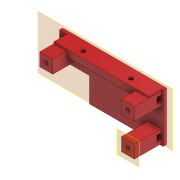
# Autodesk Inventor part: spacer for new drivetrain 2 top
Saved by Autodesk Inventor 2020 (Build 240168000, 168)
## iProperties
Created: 2020-02-19
Part Number: spacer for new drivetrain 2 top
Material: Generic
Document SubType Name: Modeling
Designer: jackm
Density: 1 g/cm^3
Appearance: Default
Author: jackm
Autodesk Inventor part; units mm, degrees
ref_plane "YZ Plane" through (0, 0, 0) normal (1, 0, 0) x (0, 1, 0)
ref_plane "XZ Plane" through (0, 0, 0) normal (0, 1, 0) x (-1, 0, 0)
ref_plane "XY Plane" through (0, 0, 0) normal (0, 0, 1) x (1, 0, 0)
ref_plane "Work Plane1" through (0, 0, 0) normal (0, 0, 1) x (1, 0, 0)
sketch "Sketch1" plane through (0, 0, 0) normal (0, 0, 1) x (1, 0, 0)
  line L0 (120, 0) -> (120, 48) construction
  line L1 (0, 48) -> (120, 48) construction
  line L2 (0, 0) -> (0, 48) construction
  line L3 (0, 0) -> (120, 0) construction
  circle A0 centre (96, 24) radius 7 construction
  circle A1 centre (72, 24) radius 7 construction
  arc A2 (88.9289, 33.8995) -> (86.1005, 31.0711) centre (87.5147, 32.4853) ccw construction
  line L4 (89.4142, 33.4142) -> (88.9289, 33.8995) construction
  arc A3 (86.5858, 30.5858) -> (89.4142, 33.4142) centre (88, 32) ccw construction
  line L5 (86.1005, 31.0711) -> (86.5858, 30.5858) construction
  line L6 (83.3137, 22) -> (84.6863, 22) construction
  arc A4 (83.3137, 26) -> (83.3137, 22) centre (83.3137, 24) ccw construction
  line L7 (84.6863, 26) -> (83.3137, 26) construction
  arc A5 (84.6863, 22) -> (84.6863, 26) centre (84.6863, 24) ccw construction
  arc A6 (86.1005, 16.9289) -> (88.9289, 14.1005) centre (87.5147, 15.5147) ccw construction
  line L8 (86.5858, 17.4142) -> (86.1005, 16.9289) construction
  arc A7 (89.4142, 14.5858) -> (86.5858, 17.4142) centre (88, 16) ccw construction
  line L9 (88.9289, 14.1005) -> (89.4142, 14.5858) construction
  arc A8 (105.8995, 31.0711) -> (103.0711, 33.8995) centre (104.4853, 32.4853) ccw construction
  line L10 (105.4142, 30.5858) -> (105.8995, 31.0711) construction
  arc A9 (102.5858, 33.4142) -> (105.4142, 30.5858) centre (104, 32) ccw construction
  line L11 (103.0711, 33.8995) -> (102.5858, 33.4142) construction
  line L12 (108.6863, 26) -> (107.3137, 26) construction
  arc A10 (108.6863, 22) -> (108.6863, 26) centre (108.6863, 24) ccw construction
  line L13 (107.3137, 22) -> (108.6863, 22) construction
  arc A11 (107.3137, 26) -> (107.3137, 22) centre (107.3137, 24) ccw construction
  line L14 (98, 35.3137) -> (98, 40) construction
  arc A12 (94, 35.3137) -> (98, 35.3137) centre (96, 35.3137) ccw construction
  line L15 (94, 40) -> (94, 35.3137) construction
  arc A13 (98, 40) -> (94, 40) centre (96, 40) ccw construction
  circle A14 centre (88, 40) radius 2 construction
  circle A15 centre (80, 40) radius 2 construction
  line L16 (74, 35.3137) -> (74, 40) construction
  arc A16 (70, 35.3137) -> (74, 35.3137) centre (72, 35.3137) ccw construction
  line L17 (70, 40) -> (70, 35.3137) construction
  arc A17 (74, 40) -> (70, 40) centre (72, 40) ccw construction
  circle A18 centre (64, 40) radius 2 construction
  circle A19 centre (56, 40) radius 2 construction
  line L18 (50, 35.3137) -> (50, 40) construction
  arc A20 (46, 35.3137) -> (50, 35.3137) centre (48, 35.3137) ccw construction
  line L19 (46, 40) -> (46, 35.3137) construction
  arc A21 (50, 40) -> (46, 40) centre (48, 40) ccw construction
  circle A22 centre (40, 40) radius 2 construction
  circle A23 centre (32, 40) radius 2 construction
  line L20 (26, 35.3137) -> (26, 40) construction
  arc A24 (22, 35.3137) -> (26, 35.3137) centre (24, 35.3137) ccw construction
  line L21 (22, 40) -> (22, 35.3137) construction
  arc A25 (26, 40) -> (22, 40) centre (24, 40) ccw construction
  circle A26 centre (16, 40) radius 2 construction
  circle A27 centre (8, 40) radius 2 construction
  line L22 (94, 12.6863) -> (94, 8) construction
  arc A28 (98, 12.6863) -> (94, 12.6863) centre (96, 12.6863) ccw construction
  line L23 (98, 8) -> (98, 12.6863) construction
  arc A29 (94, 8) -> (98, 8) centre (96, 8) ccw construction
  circle A30 centre (88, 8) radius 2 construction
  circle A31 centre (80, 8) radius 2 construction
  line L24 (70, 12.6863) -> (70, 8) construction
  arc A32 (74, 12.6863) -> (70, 12.6863) centre (72, 12.6863) ccw construction
  line L25 (74, 8) -> (74, 12.6863) construction
  arc A33 (70, 8) -> (74, 8) centre (72, 8) ccw construction
  circle A34 centre (64, 8) radius 2 construction
  circle A35 centre (56, 8) radius 2 construction
  line L26 (46, 12.6863) -> (46, 8) construction
  arc A36 (50, 12.6863) -> (46, 12.6863) centre (48, 12.6863) ccw construction
  line L27 (50, 8) -> (50, 12.6863) construction
  arc A37 (46, 8) -> (50, 8) centre (48, 8) ccw construction
  circle A38 centre (40, 8) radius 2 construction
  circle A39 centre (32, 8) radius 2 construction
  line L28 (22, 12.6863) -> (22, 8) construction
  arc A40 (26, 12.6863) -> (22, 12.6863) centre (24, 12.6863) ccw construction
  line L29 (26, 8) -> (26, 12.6863) construction
  arc A41 (22, 8) -> (26, 8) centre (24, 8) ccw construction
  circle A42 centre (16, 8) radius 2 construction
  circle A43 centre (8, 8) radius 2 construction
  arc A44 (9.8995, 31.0711) -> (7.0711, 33.8995) centre (8.4853, 32.4853) ccw construction
  line L30 (9.4142, 30.5858) -> (9.8995, 31.0711) construction
  arc A45 (6.5858, 33.4142) -> (9.4142, 30.5858) centre (8, 32) ccw construction
  line L31 (7.0711, 33.8995) -> (6.5858, 33.4142) construction
  arc A46 (7.0711, 14.1005) -> (9.8995, 16.9289) centre (8.4853, 15.5147) ccw construction
  line L32 (6.5858, 14.5858) -> (7.0711, 14.1005) construction
  arc A47 (9.4142, 17.4142) -> (6.5858, 14.5858) centre (8, 16) ccw construction
  line L33 (9.8995, 16.9289) -> (9.4142, 17.4142) construction
  arc A48 (112.9289, 33.8995) -> (110.1005, 31.0711) centre (111.5147, 32.4853) ccw construction
  line L34 (113.4142, 33.4142) -> (112.9289, 33.8995) construction
  arc A49 (110.5858, 30.5858) -> (113.4142, 33.4142) centre (112, 32) ccw construction
  line L35 (110.1005, 31.0711) -> (110.5858, 30.5858) construction
  arc A50 (110.1005, 16.9289) -> (112.9289, 14.1005) centre (111.5147, 15.5147) ccw construction
  line L36 (110.5858, 17.4142) -> (110.1005, 16.9289) construction
  arc A51 (113.4142, 14.5858) -> (110.5858, 17.4142) centre (112, 16) ccw construction
  line L37 (112.9289, 14.1005) -> (113.4142, 14.5858) construction
  circle A52 centre (104, 8) radius 2 construction
  circle A53 centre (104, 40) radius 2 construction
  circle A54 centre (112, 40) radius 2 construction
  circle A55 centre (112, 8) radius 2 construction
  arc A56 (33.8995, 31.0711) -> (31.0711, 33.8995) centre (32.4853, 32.4853) ccw construction
  line L38 (33.4142, 30.5858) -> (33.8995, 31.0711) construction
  arc A57 (30.5858, 33.4142) -> (33.4142, 30.5858) centre (32, 32) ccw construction
  line L39 (31.0711, 33.8995) -> (30.5858, 33.4142) construction
  arc A58 (57.8995, 31.0711) -> (55.0711, 33.8995) centre (56.4853, 32.4853) ccw construction
  line L40 (57.4142, 30.5858) -> (57.8995, 31.0711) construction
  arc A59 (54.5858, 33.4142) -> (57.4142, 30.5858) centre (56, 32) ccw construction
  line L41 (55.0711, 33.8995) -> (54.5858, 33.4142) construction
  arc A60 (81.8995, 31.0711) -> (79.0711, 33.8995) centre (80.4853, 32.4853) ccw construction
  line L42 (81.4142, 30.5858) -> (81.8995, 31.0711) construction
  arc A61 (78.5858, 33.4142) -> (81.4142, 30.5858) centre (80, 32) ccw construction
  line L43 (79.0711, 33.8995) -> (78.5858, 33.4142) construction
  arc A62 (14.1005, 16.9289) -> (16.9289, 14.1005) centre (15.5147, 15.5147) ccw construction
  line L44 (14.5858, 17.4142) -> (14.1005, 16.9289) construction
  arc A63 (17.4142, 14.5858) -> (14.5858, 17.4142) centre (16, 16) ccw construction
  line L45 (16.9289, 14.1005) -> (17.4142, 14.5858) construction
  arc A64 (38.1005, 16.9289) -> (40.9289, 14.1005) centre (39.5147, 15.5147) ccw construction
  line L46 (38.5858, 17.4142) -> (38.1005, 16.9289) construction
  arc A65 (41.4142, 14.5858) -> (38.5858, 17.4142) centre (40, 16) ccw construction
  line L47 (40.9289, 14.1005) -> (41.4142, 14.5858) construction
  arc A66 (62.1005, 16.9289) -> (64.9289, 14.1005) centre (63.5147, 15.5147) ccw construction
  line L48 (62.5858, 17.4142) -> (62.1005, 16.9289) construction
  arc A67 (65.4142, 14.5858) -> (62.5858, 17.4142) centre (64, 16) ccw construction
  line L49 (64.9289, 14.1005) -> (65.4142, 14.5858) construction
  line L50 (11.3137, 22) -> (12.6863, 22) construction
  arc A68 (11.3137, 26) -> (11.3137, 22) centre (11.3137, 24) ccw construction
  line L51 (12.6863, 26) -> (11.3137, 26) construction
  arc A69 (12.6863, 22) -> (12.6863, 26) centre (12.6863, 24) ccw construction
  line L52 (35.3137, 22) -> (36.6863, 22) construction
  arc A70 (35.3137, 26) -> (35.3137, 22) centre (35.3137, 24) ccw construction
  line L53 (36.6863, 26) -> (35.3137, 26) construction
  arc A71 (36.6863, 22) -> (36.6863, 26) centre (36.6863, 24) ccw construction
  line L54 (59.3137, 22) -> (60.6863, 22) construction
  arc A72 (59.3137, 26) -> (59.3137, 22) centre (59.3137, 24) ccw construction
  line L55 (60.6863, 26) -> (59.3137, 26) construction
  arc A73 (60.6863, 22) -> (60.6863, 26) centre (60.6863, 24) ccw construction
  arc A74 (16.9289, 33.8995) -> (14.1005, 31.0711) centre (15.5147, 32.4853) ccw construction
  line L56 (17.4142, 33.4142) -> (16.9289, 33.8995) construction
  arc A75 (14.5858, 30.5858) -> (17.4142, 33.4142) centre (16, 32) ccw construction
  line L57 (14.1005, 31.0711) -> (14.5858, 30.5858) construction
  arc A76 (40.9289, 33.8995) -> (38.1005, 31.0711) centre (39.5147, 32.4853) ccw construction
  line L58 (41.4142, 33.4142) -> (40.9289, 33.8995) construction
  arc A77 (38.5858, 30.5858) -> (41.4142, 33.4142) centre (40, 32) ccw construction
  line L59 (38.1005, 31.0711) -> (38.5858, 30.5858) construction
  arc A78 (64.9289, 33.8995) -> (62.1005, 31.0711) centre (63.5147, 32.4853) ccw construction
  line L60 (65.4142, 33.4142) -> (64.9289, 33.8995) construction
  arc A79 (62.5858, 30.5858) -> (65.4142, 33.4142) centre (64, 32) ccw construction
  line L61 (62.1005, 31.0711) -> (62.5858, 30.5858) construction
  arc A80 (31.0711, 14.1005) -> (33.8995, 16.9289) centre (32.4853, 15.5147) ccw construction
  line L62 (30.5858, 14.5858) -> (31.0711, 14.1005) construction
  arc A81 (33.4142, 17.4142) -> (30.5858, 14.5858) centre (32, 16) ccw construction
  line L63 (33.8995, 16.9289) -> (33.4142, 17.4142) construction
  arc A82 (55.0711, 14.1005) -> (57.8995, 16.9289) centre (56.4853, 15.5147) ccw construction
  line L64 (54.5858, 14.5858) -> (55.0711, 14.1005) construction
  arc A83 (57.4142, 17.4142) -> (54.5858, 14.5858) centre (56, 16) ccw construction
  line L65 (57.8995, 16.9289) -> (57.4142, 17.4142) construction
  arc A84 (79.0711, 14.1005) -> (81.8995, 16.9289) centre (80.4853, 15.5147) ccw construction
  line L66 (78.5858, 14.5858) -> (79.0711, 14.1005) construction
  arc A85 (81.4142, 17.4142) -> (78.5858, 14.5858) centre (80, 16) ccw construction
  line L67 (81.8995, 16.9289) -> (81.4142, 17.4142) construction
  arc A86 (103.0711, 14.1005) -> (105.8995, 16.9289) centre (104.4853, 15.5147) ccw construction
  line L68 (102.5858, 14.5858) -> (103.0711, 14.1005) construction
  arc A87 (105.4142, 17.4142) -> (102.5858, 14.5858) centre (104, 16) ccw construction
  line L69 (105.8995, 16.9289) -> (105.4142, 17.4142) construction
  circle A88 centre (24, 24) radius 7 construction
  circle A89 centre (48, 24) radius 7 construction
  line L70 (120, 0) -> (48, 0)
  line L71 (18.4, 19.8) -> (18.4, 48)
  line L72 (18.4, 48) -> (120, 48)
  line L73 (120, 0) -> (120, 48)
  line L74 (18.4, 24) -> (48, 24)
  line L75 (48, 24) -> (48, 0)
  point P0 (18.4, 0)
  dimension "d0" = 101.6
  constraints: 12 end point, 4 perpendicular, 3 point on line, 1 collinear, 2 other
  measures "d0" distance of L0.start point (18.4, 0)
extrude "Extrusion1" add sketch "Sketch1" along normal blind 3.175
ref_plane "Work Plane2" through (112, 8, 29.6672) normal (0, 0, 1) x (1, 0, 0)
sketch "Sketch5" plane through (112, 8, 29.6672) normal (0, 0, 1) x (1, 0, 0)
  circle A0 centre (0, 0) radius 3.81 construction
  circle A1 centre (0, 32) radius 3.81 construction
  circle A2 centre (-80, 32) radius 3.81 construction
  circle A3 centre (-80, 0) radius 3.81 construction
  circle A4 centre (0, 0) radius 1.9304
  circle A5 centre (0, 32) radius 1.9304
  circle A6 centre (-80, 0) radius 1.9304
  circle A7 centre (-80, 32) radius 1.9304
  point P0 (-112, -8)
  dimension "d25" = 3.8608
  dimension "d26" = 3.8608
  dimension "d27" = 3.8608
  dimension "d28" = 3.8608
  constraints: 4 centre point, 4 coincident
  measures "d25" diameter of A4
  measures "d26" diameter of A5
  measures "d27" diameter of A6
  measures "d28" diameter of A7
extrude "Extrusion4" cut sketch "Sketch5" against normal through all
sketch "Sketch6" plane through (0, 0, 3.175) normal (0, 0, 1) x (1, 0, 0)
  circle A0 centre (112, 40) radius 1.9304 projected
  line L0 (120, 0) -> (120, 48) projected
  line L1 (112, 42.9845) -> (124.5106, 42.9845) construction
  line L2 (112, 37.0028) -> (120.8332, 37.0028) construction
  line L3 (112, 40) -> (108.547, 40.0987)
  line L4 (108.547, 40.0987) -> (109.8492, 37.8432)
  line L5 (108.547, 40.0987) -> (111.1514, 40.0987) construction
  line L6 (109.8492, 37.8432) -> (110.3344, 37.0028)
  line L7 (108.547, 40.0987) -> (110.2132, 42.9845)
  line L8 (108.547, 40.0987) -> (114.1138, 40.0987) construction
  line L9 (110.2132, 42.9845) -> (118.2904, 42.9845)
  line L10 (110.3344, 37.0028) -> (118.2904, 37.0028)
  line L11 (118.2904, 46.3436) -> (105.5904, 46.3436)
  line L12 (105.5904, 46.3436) -> (105.5904, 33.6436)
  line L13 (105.5904, 33.6436) -> (118.2904, 33.6436)
  line L14 (118.2904, 33.6436) -> (118.2904, 37.0028)
  line L15 (118.2904, 46.3436) -> (118.2904, 42.9845)
  circle A1 centre (112, 8) radius 1.9304 construction
  line L16 (112, 10.9845) -> (124.5106, 10.9845) construction
  line L17 (112, 5.0028) -> (120.8332, 5.0028) construction
  line L18 (112, 8) -> (108.547, 8.0987)
  line L19 (108.547, 8.0987) -> (109.8492, 5.8432)
  line L20 (108.547, 8.0987) -> (111.1514, 8.0987) construction
  line L21 (109.8492, 5.8432) -> (110.3344, 5.0028)
  line L22 (108.547, 8.0987) -> (110.2132, 10.9845)
  line L23 (108.547, 8.0987) -> (114.1138, 8.0987) construction
  line L24 (110.2132, 10.9845) -> (118.2904, 10.9845)
  line L25 (110.3344, 5.0028) -> (118.2904, 5.0028)
  line L26 (118.2904, 14.3436) -> (105.5904, 14.3436)
  line L27 (105.5904, 14.3436) -> (105.5904, 1.6436)
  line L28 (105.5904, 1.6436) -> (118.2904, 1.6436)
  line L29 (118.2904, 1.6436) -> (118.2904, 5.0028)
  line L30 (118.2904, 14.3436) -> (118.2904, 10.9845)
  circle A2 centre (32, 40) radius 1.9304 construction
  line L31 (32.0099, 37.0155) -> (19.4993, 36.974) construction
  line L32 (31.9901, 42.9972) -> (23.1569, 42.9679) construction
  line L33 (32, 40) -> (35.4533, 39.9128)
  line L34 (35.4533, 39.9128) -> (34.1437, 42.1639)
  line L35 (35.4533, 39.9128) -> (32.849, 39.9042) construction
  line L36 (34.1437, 42.1639) -> (33.6557, 43.0027)
  line L37 (35.4533, 39.9128) -> (33.7967, 37.0214)
  line L38 (35.4533, 39.9128) -> (29.8865, 39.8943) construction
  line L39 (33.7967, 37.0214) -> (25.7196, 36.9947)
  line L40 (33.6557, 43.0027) -> (25.6997, 42.9763)
  line L41 (25.7307, 33.6355) -> (38.4306, 33.6776)
  line L42 (38.4306, 33.6776) -> (38.3885, 46.3776)
  line L43 (38.3885, 46.3776) -> (25.6886, 46.3355)
  line L44 (25.6886, 46.3355) -> (25.6997, 42.9763)
  line L45 (25.7307, 33.6355) -> (25.7196, 36.9947)
  point P0 (0, 0)
  dimension "d32" = 2.9845
  dimension "d33" = 2.9972
  dimension "d36" = 3.4544
  dimension "d37" = 60
  dimension "d38" = 60
  dimension "d39" = 8.0772
  dimension "d41" = 12.7
  dimension "d42" = 12.7
  dimension "d43" = 12.7
  dimension "d44" = 2.9845
  dimension "d45" = 2.9972
  dimension "d46" = 3.4544
  dimension "d47" = 60
  dimension "d48" = 60
  dimension "d49" = 8.0772
  dimension "d50" = 12.7
  dimension "d51" = 12.7
  dimension "d52" = 12.7
  dimension "d69" = 2.9845
  dimension "d70" = 2.9972
  dimension "d71" = 3.4544
  dimension "d72" = 60
  dimension "d73" = 60
  dimension "d74" = 8.0772
  dimension "d75" = 12.7
  dimension "d76" = 12.7
  dimension "d77" = 12.7
  constraints: 90 end point, 9 point on line, 8 horizontal, 6 perpendicular, 3 equal length
  measures "d32" distance of L3.start L1.start
  measures "d33" distance of L3.start L2.start
  measures "d36" distance of L3.start L3.end
  measures "d37" angle of L4 L5
  measures "d38" angle of L8 L7
  measures "d39" distance of L7.end L9.end
  measures "d41" distance of L11.start L11.end
  measures "d42" distance of L11.end L12.end
  measures "d43" distance of L12.end L13.end
  measures "d44" distance of L18.start L16.start
  measures "d45" distance of L18.start L17.start
  measures "d46" distance of L18.start L23.start
  measures "d47" angle of L19 L20
  measures "d48" angle of L23 L22
  measures "d49" distance of L22.end L30.end
  measures "d50" distance of L26.start L27.start
  measures "d51" distance of L27.start L28.start
  measures "d52" distance of L28.start L28.end
  measures "d69" distance of L33.start L31.start
  measures "d70" distance of L33.start L32.start
  measures "d71" distance of L33.start L35.start
  measures "d72" angle of L34 L35
  measures "d73" angle of L38 L37
  measures "d74" distance of L37.end L39.end
  measures "d75" distance of L45.start L41.end
  measures "d76" distance of L41.end L43.start
  measures "d77" distance of L43.start L43.end
extrude "Extrusion5" add sketch "Sketch6" along normal blind 4.3942 contours L4 L6 L10 L14 L13 L12 L11 L15 L9 L7 | L19 L21 L25 L29 L28 L27 L26 L30 L24 L22 | L34 L36 L40 L44 L43 L42 L41 L45 L39 L37
sketch "Sketch7" plane through (0, 0, 7.5692) normal (0, 0, 1) x (1, 0, 0)
  line L0 (105.5904, 33.6436) -> (105.5904, 46.3436) projected
  line L1 (118.2904, 46.3436) -> (118.2904, 42.9845) projected
  line L2 (105.5904, 46.3436) -> (118.2904, 46.3436)
  line L3 (118.2904, 37.0028) -> (118.2904, 33.6436) projected
  line L4 (118.2904, 46.3436) -> (118.2904, 33.6436)
  line L5 (118.2904, 33.6436) -> (105.5904, 33.6436) projected
  line L6 (118.2904, 33.6436) -> (105.5904, 33.6436)
  line L7 (105.5904, 33.6436) -> (105.5904, 46.3436)
  line L8 (105.5904, 14.3436) -> (105.5904, 1.6436) projected
  line L9 (118.2904, 14.3436) -> (118.2904, 10.9845) projected
  line L10 (105.5904, 14.3436) -> (118.2904, 14.3436)
  line L11 (118.2904, 14.3436) -> (118.2904, 1.6436)
  line L12 (105.5904, 1.6436) -> (118.2904, 1.6436) projected
  line L13 (118.2904, 1.6436) -> (105.5904, 1.6436)
  line L14 (105.5904, 1.6436) -> (105.5904, 14.3436)
  line L15 (25.6886, 46.3355) -> (38.3885, 46.3776) projected
  line L16 (38.4306, 33.6776) -> (38.3885, 46.3776) projected
  line L17 (25.6886, 46.3355) -> (38.3885, 46.3776)
  line L18 (38.3885, 46.3776) -> (38.4306, 33.6776)
  line L19 (38.4306, 33.6776) -> (25.7307, 33.6355) projected
  line L20 (38.4306, 33.6776) -> (25.7307, 33.6355)
  line L21 (25.6886, 46.3355) -> (25.6997, 42.9763) projected
  line L22 (25.7307, 33.6355) -> (25.6886, 46.3355)
  point P0 (0, 0)
  point P1 (25.6487, 46.2826)
  point P2 (25.6642, 33.5826)
  point P3 (38.3487, 46.2981)
  point P4 (38.3642, 33.5981)
  constraints: 24 end point, 5 perpendicular, 4 collinear, 2 horizontal
extrude "Extrusion6" add sketch "Sketch7" along normal blind 22.098
sketch "Sketch8" plane through (0, 0, 29.6672) normal (0, 0, 1) x (1, 0, 0)
  circle A0 centre (32, 40) radius 1.9304 construction
  circle A1 centre (112, 40) radius 1.9304 construction
  circle A2 centre (112, 8) radius 1.9304 construction
  circle A3 centre (32, 40) radius 1.9304 projected
  circle A4 centre (32, 40) radius 1.9304
  circle A5 centre (112, 40) radius 1.9304 projected
  circle A6 centre (112, 40) radius 1.9304
  circle A7 centre (112, 8) radius 1.9304 projected
  circle A8 centre (112, 8) radius 1.9304
  point P0 (0, 0)
  constraints: 3 centre point, 3 coincident
extrude "Extrusion7" cut sketch "Sketch8" against normal through all
sketch "Sketch9" plane through (18.4, 48, 0) normal (0, 1, 0) x (1, 0, 0)
  line L0 (7.3196, -3.175) -> (7.3196, -7.5692) projected
  line L1 (99.8904, -3.175) -> (99.8904, -29.6672) projected
  line L2 (7.3196, -3.175) -> (99.8904, -3.175)
  line L3 (99.8904, -3.175) -> (99.8904, -15.875)
  line L4 (99.8904, -15.875) -> (7.3196, -15.875)
  line L5 (7.3196, -15.875) -> (7.3196, -3.175)
  point P0 (-18.4, 0)
  point P1 (7.3196, -7.5692)
  dimension "d78" = 12.7
  constraints: 8 end point, 2 parallel, 1 horizontal, 1 perpendicular, 1 point on line
  measures "d78" distance of L2.end L3.end
extrude "Extrusion8" add sketch "Sketch9" against normal up to surface surface through (38.3885, 46.3776, 3.175) normal (-0.0033161, 0.9999945, 0)
sketch "Sketch10" plane through (38.3885, 46.3776, 3.175) normal (0.0033161, -0.9999945, 0) x (0.9999945, 0.0033161, 0)
  line L0 (79.9023, 12.7) -> (0, 12.7) projected
  line L1 (67.1592, 0) -> (67.1592, 26.4922) projected
  line L2 (0, 12.7) -> (67.1592, 12.7)
  line L3 (67.1592, 12.7) -> (67.1592, 0)
  line L4 (67.1592, 0) -> (0, 0)
  line L5 (0, 0) -> (0, 12.7)
  point P0 (-38.5421, -3.175)
  constraints: 8 end point, 2 parallel, 1 horizontal, 1 perpendicular
extrude "Extrusion9" add sketch "Sketch10" along normal blind 5.08
sketch "Sketch11" plane through (38.4054, 41.2976, 3.175) normal (0.0033161, -0.9999945, 0) x (0.9999945, 0.0033161, 0)
  circle A0 centre (9.632, 6.2821) radius 4.6609 construction
  line L0 (14.2929, 6.2821) -> (11.9624, 10.3186)
  line L1 (11.9624, 10.3186) -> (7.3015, 10.3186)
  line L2 (7.3015, 10.3186) -> (4.9711, 6.2821)
  line L3 (4.9711, 6.2821) -> (7.3015, 2.2456)
  line L4 (7.3015, 2.2456) -> (11.9624, 2.2456)
  line L5 (11.9624, 2.2456) -> (14.2929, 6.2821)
  circle A1 centre (56.3463, 6.2821) radius 4.6609 construction
  line L6 (54.0158, 2.2456) -> (58.6767, 2.2456)
  line L7 (58.6767, 2.2456) -> (61.0072, 6.2821)
  line L8 (51.6854, 6.2821) -> (54.0158, 2.2456)
  line L9 (61.0072, 6.2821) -> (58.6767, 10.3186)
  line L10 (58.6767, 10.3186) -> (54.0158, 10.3186)
  line L11 (54.0158, 10.3186) -> (51.6854, 6.2821)
  point P0 (-38.5421, -3.175)
  constraints: 24 end point, 2 horizontal alignment, 2 other
extrude "Extrusion10" cut sketch "Sketch11" against normal blind 5.08
sketch "Sketch13" plane through (38.3885, 46.3776, 3.175) normal (0.0033161, -0.9999945, 0) x (0.9999945, 0.0033161, 0)
  circle A0 centre (56.3463, 6.2821) radius 1.9304
  circle A1 centre (9.632, 6.2821) radius 1.9304
  point P0 (-38.5421, -3.175)
  dimension "d85" = 3.8608
  dimension "d86" = 3.8608
  constraints: 2 centre point
  measures "d85" diameter of A0
  measures "d86" diameter of A1
extrude "Extrusion11" cut sketch "Sketch13" against normal through all
fillet "Fillet4" radius 3.175 1 edges at (71.9848, 41.409, 3.175)
body "Solid1"
